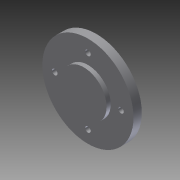
# Autodesk Inventor part: wheel hub
Saved by Autodesk Inventor 2012 (Build 160160000, 160)
## iProperties
Created: 2011-12-01
Part Number: wheel hub
Material: Default
Document SubType Name: Modeling
Designer: Antonella
Density: 1 g/cm^3
Author: Antonella
Autodesk Inventor part; units mm, degrees
ref_plane "YZ Plane" through (0, 0, 0) normal (1, 0, 0) x (0, 1, 0)
ref_plane "XZ Plane" through (0, 0, 0) normal (0, 1, 0) x (-1, 0, 0)
ref_plane "XY Plane" through (0, 0, 0) normal (0, 0, 1) x (1, 0, 0)
sketch "Sketch1" plane through (0, 0, 0) normal (0, 0, 1) x (1, 0, 0)
  line L0 (-97.79, 0) -> (97.79, 0) projected
  line L1 (0, -97.79) -> (0, 97.79) projected
  circle A0 centre (0, 0) radius 69.85
  circle A1 centre (0, 0) radius 50.8 construction
  dimension "d0" = 101.6
  dimension "d1" = 139.7
  constraints: 2 centre point, 2 coincident
  measures "d0" diameter of A1
  measures "d1" diameter of A0
extrude "Extrusion1" add sketch "Sketch1" along normal blind 12.7
sketch "Sketch2" plane through (0, 0, 12.7) normal (0, 0, 1) x (1, 0, 0)
  circle A0 centre (0, 0) radius 69.85 projected
  circle A1 centre (0, 0) radius 34.925
  dimension "d4" = 69.85
  constraints: 1 centre point, 1 coincident
  measures "d4" diameter of A1
extrude "Extrusion2" add sketch "Sketch2" along normal blind 6.35 contours A1
sketch "Sketch3" plane through (0, 0, 12.7) normal (0, 0, 1) x (1, 0, 0)
  circle A0 centre (0, 0) radius 34.925 projected
  circle A1 centre (0, 0) radius 69.85 projected
  line L0 (-97.79, 0) -> (97.79, 0) projected
  line L1 (0, -97.79) -> (0, 97.79) projected
  circle A2 centre (0, 0) radius 50.8 construction
  point P0 (0, 50.8)
  point P1 (-50.8, 0)
  point P2 (0, -50.8)
  point P3 (50.8, 0)
  dimension "d8" = 101.6
  dimension "d11" = 360
  constraints: 1 coincident, 1 point on line, 1 vertical alignment, 7 other
hole "Hole1" at (0, 50.8, 12.7) at (-50.8, 0, 12.7) at (0, -50.8, 12.7) at (50.8, 0, 12.7) direction (0, 0, -1) diameter 8.4328 end through all clearance for "Flat Head Machine Screw (82)" size "5/16" standard "Ansi Unified Screw Threads"
body "Solid1"
